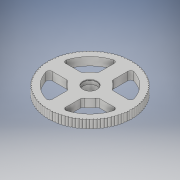
# Autodesk Inventor part: Rotator
Saved by Autodesk Inventor 2019.4 (Build 234330000, 330)
## iProperties
Created: 2019-12-23
Part Number: Rotator
Material: Generic
Document SubType Name: Modeling
Designer: Jorian Bruslind
Density: 1 g/cm^3
Appearance: Default
Author: Jorian Bruslind
Autodesk Inventor part; units mm, degrees
ref_plane "YZ Plane" through (0, 0, 0) normal (1, 0, 0) x (0, 1, 0)
ref_plane "XZ Plane" through (0, 0, 0) normal (0, 1, 0) x (-1, 0, 0)
ref_plane "XY Plane" through (0, 0, 0) normal (0, 0, 1) x (1, 0, 0)
sketch "Sketch1" plane through (0, 0, 0) normal (0, 1, 0) x (-1, 0, 0)
  circle A0 centre (0, 0) radius 15
  dimension "d0" = 30
  constraints: 1 centre point, 1 coincident
  measures "d0" diameter of A0
extrude "Extrusion1" add sketch "Sketch1" along normal blind 3
sketch "Sketch2" plane through (0, 3, 0) normal (0, 1, 0) x (1, 0, 0)
  point P0 (0, 0)
  point P1 (0, 0)
  constraints: 1 coincident
hole "Hole1" at (0, 3, 0) direction (0, -1, 0) diameter 5.1 depth 1.5 tip angle 118 counterbore diameter 5.31 counterbore depth 0.25
sketch "Sketch3" plane through (0, 3, 0) normal (0, 1, 0) x (1, 0, 0)
  arc A0 (12.754, 2.5169) -> (2.5, 12.7574) centre (0, 0) ccw
  arc A1 (-2.5169, 12.754) -> (-12.7574, 2.5) centre (0, 0) ccw
  arc A2 (-12.754, -2.5169) -> (-2.5, -12.7574) centre (0, 0) ccw
  arc A3 (2.5169, -12.754) -> (12.7574, -2.5) centre (0, 0) ccw
  arc A4 (5.4466, 2.5169) -> (2.5, 5.4544) centre (0, 0) ccw
  arc A5 (-2.5169, 5.4466) -> (-5.4544, 2.5) centre (0, 0) ccw
  arc A6 (-5.4466, -2.5169) -> (-2.5, -5.4544) centre (0, 0) ccw
  arc A7 (2.5169, -5.4466) -> (5.4544, -2.5) centre (0, 0) ccw
  line L0 (5.4466, 2.5169) -> (12.754, 2.5169)
  line L1 (2.5, 12.7574) -> (2.5, 5.4544)
  line L2 (-12.7574, 2.5) -> (-5.4544, 2.5)
  line L3 (-2.5169, 5.4466) -> (-2.5169, 12.754)
  line L4 (-2.5, -12.7574) -> (-2.5, -5.4544)
  line L5 (-5.4466, -2.5169) -> (-12.754, -2.5169)
  line L6 (12.7574, -2.5) -> (5.4544, -2.5)
  line L7 (2.5169, -5.4466) -> (2.5169, -12.754)
  dimension "d17" = 360
  dimension "d22" = 360
  dimension "d26" = 360
  constraints: 16 end point, 16 point on circle, 8 centre point, 1 coincident, 59 other
extrude "Extrusion2" cut sketch "Sketch3" against normal blind 3 contours L0 A4 L1 A0
pattern_circular "Circular Pattern1" count 4 over 360 about axis through (0, 2.25, 0) along (0, 1, 0) of "Extrusion2"
fillet "Fillet1" radius 1 4 edges at (2.5, 1.5, -12.7574) (12.754, 1.5, -2.5169) (5.4466, 1.5, -2.5169) (2.5, 1.5, -5.4544)
pattern_circular "Circular Pattern2" count 4 over 360 about axis through (0, 2.875, 0) along (0, 1, 0) of "Fillet1"
sketch "Sketch4" plane through (0, 0, 0) normal (0, -1, 0) x (1, 0, 0)
  line L0 (0, 0) -> (-15, 0)
  line L1 (0, 0) -> (15, 0) construction
  circle A0 centre (-15, 0) radius 0.5
  dimension "d37" = 15
  dimension "d38" = 180
  dimension "d39" = 1
  constraints: 4 end point, 2 horizontal, 1 centre point, 1 coincident, 1 collinear
  measures "d37" distance of L0.start L0.end
  measures "d38" angle of L0 L1
  measures "d39" diameter of A0
extrude "Extrusion3" add sketch "Sketch4" against normal blind 3
pattern_circular "Circular Pattern3" count 100 over 360 about axis through (0, 2.25, 0) along (0, 1, 0) of "Extrusion3"
body "Solid1"
